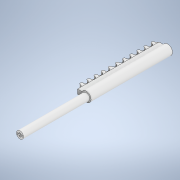
# Autodesk Inventor part: Rack
Saved by Autodesk Inventor 2020 (Build 240168000, 168)
## iProperties
Created: 2021-06-18
Part Number: Rack
Material: PVC-Piping
Document SubType Name: Modeling
Designer: ugwue
Density: 1.4 g/cm^3
Appearance: Smooth - White
Author: ugwue
Autodesk Inventor part; units mm, degrees
ref_plane "YZ Plane" through (0, 0, 0) normal (1, 0, 0) x (0, 1, 0)
ref_plane "XZ Plane" through (0, 0, 0) normal (0, 1, 0) x (-1, 0, 0)
ref_plane "XY Plane" through (0, 0, 0) normal (0, 0, 1) x (1, 0, 0)
sketch "Sketch4" plane through (0, 0, 0) normal (0, 0, 1) x (1, 0, 0)
  arc A0 (-4.1833, -2.25) -> (-4.1833, 2.25) centre (0, 0) ccw
  line L0 (-4.1833, 2.25) -> (-10, 2.25)
  line L1 (-10, 2.25) -> (-10, -2.25)
  line L2 (-10, -2.25) -> (-4.1833, -2.25)
  line L3 (10, 2.25) -> (-10, -2.25) construction
  line L4 (10, -2.25) -> (4.634146, -1.042683) construction
  line L5 (0, 0) -> (-10, 2.25) construction
  constraints: 12 end point, 3 point on circle, 2 midpoint, 1 centre point, 1 coincident, 1 parallel
extrude "Extrusion4" add sketch "Sketch4" along normal blind 80
sketch "Sketch5" plane through (0, 0, 80) normal (0, 0, 1) x (1, 0, 0)
  circle A0 centre (0, 0) radius 3.5
  dimension "d22" = 7
  constraints: 1 centre point, 1 coincident
  measures "d22" diameter of A0
extrude "Extrusion5" add sketch "Sketch5" along normal blind 65
sketch "Sketch6" plane through (0, 0, 0) normal (0, 0, -1) x (-1, 0, 0)
  point P0 (0, 0)
sketch "Sketch7" plane through (0, 0, 145) normal (0, 0, 1) x (1, 0, 0)
  line L0 (2.575, 0.8) -> (2.575, -0.8)
  line L1 (-2.575, -0.8) -> (-2.575, 0.8)
  line L2 (-2.575, 0.8) -> (2.575, -0.8) construction
  line L3 (2.575, 0.8) -> (-2.575, -0.8) construction
  line L4 (-0.8, -1.575) -> (0.8, -1.575)
  line L5 (0.8, 1.575) -> (-0.8, 1.575)
  line L6 (-0.8, -1.575) -> (0.8, 1.575) construction
  line L7 (0.8, -1.575) -> (-0.8, 1.575) construction
  line L8 (-2.575, 0.8) -> (-0.8, 0.8)
  line L9 (0.8, 0.8) -> (2.575, 0.8)
  line L10 (2.575, -0.8) -> (0.8, -0.8)
  line L11 (-0.8, -0.8) -> (-2.575, -0.8)
  line L12 (-0.8, 1.575) -> (-0.8, 0.8)
  line L13 (-0.8, -0.8) -> (-0.8, -1.575)
  line L14 (0.8, -1.575) -> (0.8, -0.8)
  line L15 (0.8, 0.8) -> (0.8, 1.575)
  point P0 (0, 0)
  dimension "d25" = 5.15
  dimension "d26" = 1.6
  dimension "d27" = 1.6
  dimension "d28" = 3.15
  constraints: 32 end point, 10 parallel, 4 midpoint, 4 perpendicular, 3 horizontal
  measures "d25" distance of L1.end L0.start
  measures "d26" distance of L0.start L0.end
  measures "d27" distance of L4.start L4.end
  measures "d28" distance of L5.start L4.end
extrude "Extrusion6" cut sketch "Sketch7" against normal blind 25
sketch "Sketch8" plane through (-10, -2.25, 0) normal (0, -1, 0) x (1, 0, 0)
  line L0 (0, 80) -> (5.8167, 80) projected
  line L1 (0, 0) -> (1.5, 0)
  line L2 (1.5, 0) -> (1.5, 80)
  line L3 (1.5, 80) -> (0, 80)
  line L4 (0, 80) -> (0, 0)
  point P0 (10, 0)
  dimension "d31" = 1.5
  constraints: 8 end point, 2 parallel, 1 horizontal, 1 perpendicular, 1 point on line
  measures "d31" distance of L3.end L2.end
extrude "Extrusion7" cut sketch "Sketch8" against normal blind 4.5
sketch "Sketch10" plane through (-4.1833, 2.25, 80) normal (0, 1, 0) x (1, 0, 0)
  spline S0 degree 3 poles (-4.318185, 79.907811) (-4.366983, 79.80467) (-4.46458, 79.598387) (-4.634268, 79.300848) (-4.82122, 79.013987) (-5.027995, 78.740957) (-5.217255, 78.527197) (-5.37941, 78.366625) (-5.506638, 78.252105) (-5.639625, 78.144264) (-5.778883, 78.044768) (-5.923983, 77.95354) (-6.027114, 77.904638) (-6.078673, 77.88019) knots 0 0 0 0 0.12500428 0.25000946 0.37501176 0.50000935 0.62499976 0.68750705 0.75001332 0.81251807 0.87502033 0.93751797 1 1 1 1
  spline S1 degree 3 poles (-6.078673, 77.88019) (-6.138182, 77.886091) (-6.257204, 77.897894) (-6.436702, 77.899878) (-6.615972, 77.893464) (-6.794503, 77.874418) (-6.970677, 77.840248) (-7.144316, 77.794556) (-7.312055, 77.730428) (-7.473551, 77.651934) (-7.624749, 77.5549) (-7.763852, 77.441124) (-7.885997, 77.30913) (-7.988232, 77.161154) (-8.066818, 76.999299) (-8.118503, 76.826872) (-8.139539, 76.647939) (-8.132956, 76.468616) (-8.139539, 76.289293) (-8.118503, 76.110361) (-8.066818, 75.937933) (-7.988232, 75.776079) (-7.885997, 75.628102) (-7.763852, 75.496109) (-7.624749, 75.382333) (-7.473551, 75.285299) (-7.312055, 75.206804) (-7.144316, 75.142677) (-6.970677, 75.096985) (-6.794503, 75.062815) (-6.615972, 75.043769) (-6.436702, 75.037355) (-6.257204, 75.039338) (-6.138182, 75.051141) (-6.078673, 75.057043) knots 0 0 0 0 0.01793242 0.03586597 0.05379826 0.07173051 0.08966209 0.10759276 0.12552301 0.14344763 0.16137049 0.17929485 0.1972189 0.21513999 0.23306033 0.25097622 0.26889048 0.28682346 0.30475644 0.3226707 0.34058659 0.35850694 0.37642803 0.39435207 0.41227644 0.43019929 0.44812392 0.46605417 0.48398484 0.50191641 0.51984866 0.53778095 0.5557145 0.57364693 0.57364693 0.57364693 0.57364693
  spline S2 degree 3 poles (-6.078673, 75.057043) (-6.027114, 75.032595) (-5.923983, 74.983692) (-5.778883, 74.892465) (-5.639625, 74.792969) (-5.506638, 74.685128) (-5.37941, 74.570607) (-5.217255, 74.410035) (-5.027995, 74.196275) (-4.82122, 73.923246) (-4.634268, 73.636385) (-4.46458, 73.338846) (-4.366983, 73.132563) (-4.318185, 73.029421) knots 0 0 0 0 0.06248203 0.12497967 0.18748193 0.24998668 0.31249295 0.37500024 0.49999065 0.62498824 0.74999054 0.87499572 1 1 1 1
  line L0 (-4.318185, 73.029421) -> (-4.318185, 79.907811)
  line L1 (-4.3167, 80) -> (-4.3167, 0)
  point P0 (4.1833, 80)
  point P1 (-4.468462, 79.600368)
  point P2 (-4.637147, 79.302624)
  point P3 (-4.824528, 79.016287)
  point P4 (-5.031388, 78.743706)
  point P5 (-5.258678, 78.487936)
  point P6 (-5.380344, 78.367611)
  point P7 (-5.5076, 78.253217)
  point P8 (-5.640673, 78.145652)
  point P9 (-5.779863, 78.046142)
  point P10 (-5.925597, 77.956512)
  point P11 (-6.257361, 77.895274)
  point P12 (-6.436668, 77.898478)
  point P13 (-6.61585, 77.891358)
  point P14 (-6.794113, 77.871897)
  point P15 (-6.970258, 77.838327)
  point P16 (-7.143338, 77.791481)
  point P17 (-7.311036, 77.728025)
  point P18 (-7.471843, 77.64884)
  point P19 (-7.622729, 77.552113)
  point P20 (-7.761027, 77.438086)
  point P21 (-7.882686, 77.306457)
  point P22 (-7.984294, 77.158835)
  point P23 (-8.062341, 76.99752)
  point P24 (-8.113396, 76.825789)
  point P25 (-8.134933, 76.647946)
  point P26 (-8.135152, 76.468616)
  point P27 (-8.134933, 76.289287)
  point P28 (-8.113396, 76.111444)
  point P29 (-8.062341, 75.939713)
  point P30 (-7.984294, 75.778398)
  point P31 (-7.882686, 75.630776)
  point P32 (-7.761027, 75.499147)
  point P33 (-7.622729, 75.38512)
  point P34 (-7.471843, 75.288393)
  point P35 (-7.311036, 75.209208)
  point P36 (-7.143338, 75.145751)
  point P37 (-6.970258, 75.098906)
  point P38 (-6.794113, 75.065336)
  point P39 (-6.61585, 75.045874)
  point P40 (-6.436668, 75.038754)
  point P41 (-6.257361, 75.041959)
  point P42 (-5.925597, 74.980721)
  point P43 (-5.779863, 74.891091)
  point P44 (-5.640673, 74.79158)
  point P45 (-5.5076, 74.684016)
  point P46 (-5.380344, 74.569622)
  point P47 (-5.258678, 74.449297)
  point P48 (-5.031388, 74.193527)
  point P49 (-4.824528, 73.920946)
  point P50 (-4.637147, 73.634608)
  point P51 (-4.468462, 73.336864)
  constraints: 2 end point, 1 parallel, 57 other
sketch "Sketch10 outline for Extrusion8" plane through (-4.1833, 2.25, 80) normal (0, 1, 0) x (1, 0, 0)
  spline S0 degree 3 poles (-6.078673, 77.88019) (-6.138182, 77.886091) (-6.257204, 77.897894) (-6.436702, 77.899878) (-6.615972, 77.893464) (-6.794503, 77.874418) (-6.970677, 77.840248) (-7.144316, 77.794556) (-7.312055, 77.730428) (-7.473551, 77.651934) (-7.624749, 77.5549) (-7.763852, 77.441124) (-7.885997, 77.30913) (-7.988232, 77.161154) (-8.066818, 76.999299) (-8.118503, 76.826872) (-8.139539, 76.647939) (-8.132956, 76.468616) (-8.139539, 76.289293) (-8.118503, 76.110361) (-8.066818, 75.937933) (-7.988232, 75.776079) (-7.885997, 75.628102) (-7.763852, 75.496109) (-7.624749, 75.382333) (-7.473551, 75.285299) (-7.312055, 75.206804) (-7.144316, 75.142677) (-6.970677, 75.096985) (-6.794503, 75.062815) (-6.615972, 75.043769) (-6.436702, 75.037355) (-6.257204, 75.039338) (-6.138182, 75.051141) (-6.078673, 75.057043) knots 0 0 0 0 0.03126038 0.06252273 0.09378289 0.12504297 0.15630187 0.1875592 0.2188158 0.25006259 0.28130629 0.31255263 0.34379841 0.37503904 0.40627836 0.43750992 0.46873864 0.5 0.53126136 0.56249008 0.59372164 0.62496096 0.65620159 0.68744737 0.71869371 0.74993741 0.7811842 0.8124408 0.84369813 0.87495703 0.90621711 0.93747727 0.96873962 1 1 1 1
  spline S1 degree 3 poles (-4.318185, 79.907811) (-4.366983, 79.80467) (-4.46458, 79.598387) (-4.634268, 79.300848) (-4.82122, 79.013987) (-5.027995, 78.740957) (-5.217255, 78.527197) (-5.37941, 78.366625) (-5.506638, 78.252105) (-5.639625, 78.144264) (-5.778883, 78.044768) (-5.923983, 77.95354) (-6.027114, 77.904638) (-6.078673, 77.88019) knots 0 0 0 0 0.12500428 0.25000946 0.37501176 0.50000935 0.62499976 0.68750705 0.75001332 0.81251807 0.87502033 0.93751797 1 1 1 1
  line L0 (-4.318185, 73.029421) -> (-4.318185, 79.907811)
  spline S2 degree 3 poles (-6.078673, 75.057043) (-6.027114, 75.032595) (-5.923983, 74.983692) (-5.778883, 74.892465) (-5.639625, 74.792969) (-5.506638, 74.685128) (-5.37941, 74.570607) (-5.217255, 74.410035) (-5.027995, 74.196275) (-4.82122, 73.923246) (-4.634268, 73.636385) (-4.46458, 73.338846) (-4.366983, 73.132563) (-4.318185, 73.029421) knots 0 0 0 0 0.06248203 0.12497967 0.18748193 0.24998668 0.31249295 0.37500024 0.49999065 0.62498824 0.74999054 0.87499572 1 1 1 1
extrude "Extrusion8" add sketch "Sketch10 outline for Extrusion8" against normal blind 4.5
pattern_linear "Rectangular Pattern3" count 11 spacing 7 along (0, 0, 1) of "Extrusion8"
body "Solid2"
